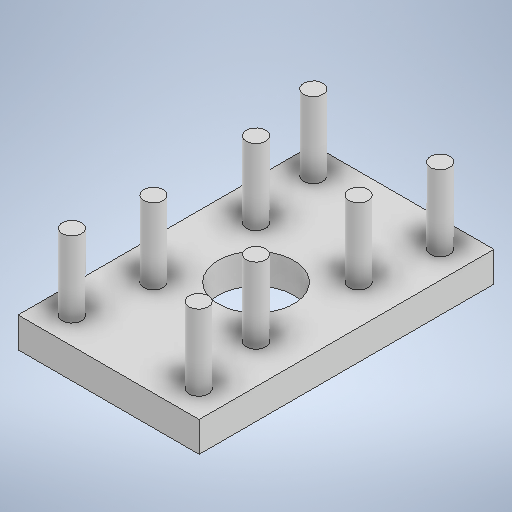
# Autodesk Inventor part: Plate
Saved by Autodesk Inventor 2027 (Build 310192060, 192F)
## iProperties
Created: 2026-07-07
Part Number: Plate
Material: Generic
Document SubType Name: Modeling
Designer: 13129
Density: 1 g/cm^3
Appearance: Default
Author: 13129
Autodesk Inventor part; units mm, degrees
ref_plane "YZ Plane" through (0, 0, 0) normal (1, 0, 0) x (0, 1, 0)
ref_plane "XZ Plane" through (0, 0, 0) normal (0, 1, 0) x (-1, 0, 0)
ref_plane "XY Plane" through (0, 0, 0) normal (0, 0, 1) x (1, 0, 0)
sketch "Sketch1" plane through (0, 0, 0) normal (0, 1, 0) x (-1, 0, 0)
  line L0 (0, 0) -> (0, -48.84)
  line L1 (0, -48.84) -> (30, -48.84)
  line L2 (30, -48.84) -> (30, 0)
  line L3 (30, 0) -> (0, 0)
  circle A0 centre (4.5, -44.42) radius 1.6
  circle A1 centre (25.5, -44.42) radius 1.6
  circle A2 centre (15, -24.42) radius 6.25
  circle A3 centre (6.5, -32.92) radius 1.6
  circle A4 centre (23.5, -32.92) radius 1.6
  circle A5 centre (6.5, -15.92) radius 1.6
  circle A6 centre (23.5, -15.92) radius 1.6
  circle A7 centre (4.5, -4.42) radius 1.6
  circle A8 centre (25.5, -4.42) radius 1.6
  line L4 (23.5, -32.92) -> (23.5, -15.92)
  line L5 (23.5, -24.42) -> (6.5, -24.42)
  line L6 (25.5, -44.42) -> (4.5, -44.42)
  line L7 (4.5, -44.42) -> (4.5, -4.42)
  point P0 (30, -24.42)
  point P1 (15, -48.84)
  point P2 (15, -24.42)
  point P3 (4.5, -24.42)
  point P4 (0, -24.42)
  point P5 (15, -44.42)
  dimension "d0" = 48.84
  dimension "d1" = 30
  dimension "d2" = 12.5
  dimension "d3" = 17
  dimension "d4" = 17
  dimension "d5" = 3.2
  dimension "d6" = 21
  dimension "d7" = 40
  constraints: 16 end point, 9 centre point, 8 vertical alignment, 7 equal radius, 7 horizontal alignment, 7 midpoint, 3 perpendicular, 3 vertical, 1 horizontal, 1 parallel
  measures "d0" distance of L0.start L0.end
  measures "d1" distance of L0.end L1.end
  measures "d2" diameter of A2
  measures "d3" distance of A3.centre L4.start
  measures "d4" distance of A5.centre A3.centre
  measures "d5" diameter of A4
  measures "d6" distance of L6.start L6.end
  measures "d7" distance of L6.end L7.end
extrude "Extrusion1" add sketch "Sketch1" along normal blind 5
sketch "Sketch2" plane through (0, 0, 0) normal (0, -1, 0) x (1, 0, 0)
  circle A0 centre (-23.5, -15.92) radius 1.6 construction
  circle A1 centre (-4.5, -4.42) radius 1.6 construction
  circle A2 centre (-25.5, -44.42) radius 1.6 construction
  circle A3 centre (-25.5, -4.42) radius 1.6 construction
  circle A4 centre (-4.5, -44.42) radius 1.6 construction
  circle A5 centre (-6.5, -32.92) radius 1.6 construction
  circle A6 centre (-23.5, -32.92) radius 1.6 construction
  circle A7 centre (-6.5, -15.92) radius 1.6 construction
  circle A8 centre (-4.5, -44.42) radius 1.6
  circle A9 centre (-6.5, -32.92) radius 1.6
  circle A10 centre (-6.5, -15.92) radius 1.6
  circle A11 centre (-4.5, -4.42) radius 1.6
  circle A12 centre (-25.5, -4.42) radius 1.6
  circle A13 centre (-23.5, -15.92) radius 1.6
  circle A14 centre (-23.5, -32.92) radius 1.6
  circle A15 centre (-25.5, -44.42) radius 1.6
  constraints: 8 centre point, 8 coincident, 8 concentric
extrude "Extrusion2" add sketch "Sketch2" against normal blind 17.5
body "Solid1"
